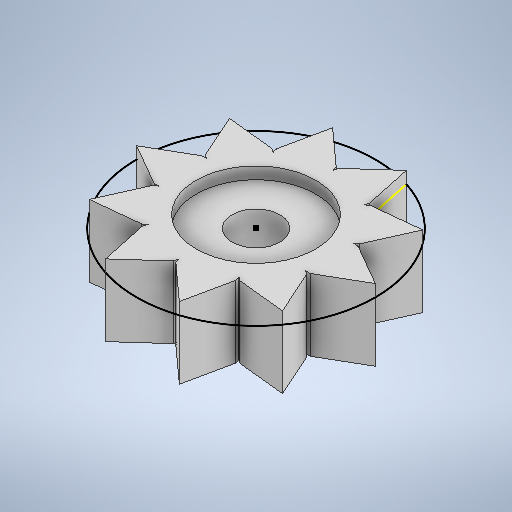
# Autodesk Inventor part: Part8
Saved by Autodesk Inventor 2025.2 (Build 292293000, 293)
## iProperties
Created: 2025-03-26
Part Number: Part8
Material: Generic
Document SubType Name: Sheet Metal
Designer: ziyuz
Density: 1 g/cm^3
Sheet Metal Rule: Default_mm
Appearance: Default
Author: ziyuz
Autodesk Inventor part; units mm, degrees
ref_plane "YZ Plane" through (0, 0, 0) normal (1, 0, 0) x (0, 1, 0)
ref_plane "XZ Plane" through (0, 0, 0) normal (0, 1, 0) x (-1, 0, 0)
ref_plane "XY Plane" through (0, 0, 0) normal (0, 0, 1) x (1, 0, 0)
sketch "Sketch1" plane through (0, 0, 0) normal (0, 1, 0) x (-1, 0, 0)
  circle A0 centre (0, 0) radius 25
  circle A1 centre (0, 0) radius 22.5
  circle A2 centre (0, 0) radius 2.25
  line L0 (10, 10) -> (-10, 10)
  line L1 (-10, 10) -> (-10, -10)
  line L2 (-10, -10) -> (10, -10)
  line L3 (10, -10) -> (10, 10)
  line L4 (10, 10) -> (-10, -10) construction
  line L5 (-10, 10) -> (10, -10) construction
  circle A3 centre (10, -10) radius 2.5
  circle A4 centre (-10, -10) radius 2.5
  circle A5 centre (-10, 10) radius 2.5
  circle A6 centre (10, 10) radius 2.5
  circle A7 centre (0, 0) radius 5
  circle A8 centre (0, 0) radius 2.5
  circle A9 centre (0, 0) radius 1
  dimension "d0" = 50
  dimension "d1" = 45
  dimension "d2" = 4.5
  dimension "d3" = 20
  dimension "d4" = 20
  dimension "d5" = 5
  dimension "d6" = 5
  dimension "d7" = 5
  dimension "d8" = 5
  dimension "d27" = 10
  dimension "d28" = 5
  dimension "d29" = 2
  constraints: 12 end point, 10 centre point, 10 coincident, 2 midpoint, 2 parallel, 1 horizontal, 1 perpendicular
  measures "d0" diameter of A0
  measures "d1" diameter of A1
  measures "d2" diameter of A2
  measures "d3" distance of L2.end L1.end
  measures "d4" distance of L1.end L0.end
  measures "d5" diameter of A3
  measures "d6" diameter of A4
  measures "d7" diameter of A5
  measures "d8" diameter of A6
  measures "d27" diameter of A7
  measures "d28" diameter of A8
  measures "d29" diameter of A9
extrude "Extrusion1" add sketch "Sketch1" along normal blind 2 contours A2 | A8
sketch "Sketch5" plane through (0, 2, 0) normal (0, 1, 0) x (1, 0, 0)
  circle A0 centre (0, 0) radius 5
  line L0 (-5, 0) -> (-3.2679, 1)
  line L1 (-5, 0) -> (-3, 0) construction
  line L2 (-3.2679, 1) -> (-2.2913, 1)
  circle A1 centre (0, 0) radius 2.5 projected
  line L3 (-5, 0) -> (-3.2679, -1)
  line L4 (-5, 0) -> (-3, 0) construction
  line L5 (-3.2679, -1) -> (-2.2913, -1)
  dimension "d30" = 10
  dimension "d31" = 2
  dimension "d32" = 30
  dimension "d33" = 2
  dimension "d34" = 30
  constraints: 12 end point, 3 horizontal, 2 equal length, 2 point on circle, 1 coincident, 1 horizontal alignment, 1 parallel, 2 other
  measures "d31" distance of L0.start L0.end
  measures "d32" angle of L1 L0
  measures "d33" distance of L0.start L3.end
  measures "d34" angle of L3 L4
extrude "Extrusion4" add sketch "Sketch5" along normal blind 0.5 and the other way blind 2.5 contours L0 L2 A1 L5 L3
pattern_circular "Circular Pattern2" count 10 over 360 about axis through (0, 0, 0) along (0, 1, 0) of "Extrusion4"
sketch "Sketch6" plane through (0, 2, 0) normal (0, 1, 0) x (1, 0, 0)
  line L0 (1.5451, 4.7553) -> (1.9609, 2.799) projected
  circle A0 centre (0, 0) radius 5
  constraints: 1 coincident, 3 other
equation "\"BendRadius\" = Thickness"
equation "\"BendReliefWidth\" = Thickness"
equation "\"BendReliefDepth\" = 0.5 * Thickness"
equation "\"CornerReliefSize\" = 4 * Thickness"
equation "\"MinimumRemnant\" = 2 * Thickness"
equation "\"TransitionRadius\" = BendRadius"
equation "\"JacobiRadiusSize\" = BendRadius"
equation "\"GapSize\" = Thickness"
equation "\"Thickness\" = 0.5"
body "Solid1"
